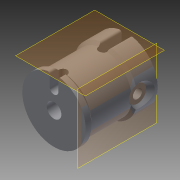
# Autodesk Inventor part: PULLEY
Saved by Autodesk Inventor 2013 (Build 170138000, 138)
## iProperties
Created: 2013-12-16
Part Number: PULLEY
Material: Generic
Document SubType Name: Modeling
Designer: employee
Density: 1 g/cm^3
Author: employee
Autodesk Inventor part; units mm, degrees
ref_plane "XY Plane" through (0, 0, 0) normal (0, 0, 1) x (1, 0, 0)
sketch "Sketch1" plane through (0, 0, 0) normal (0, 0, 1) x (1, 0, 0)
  circle A0 centre (0, 0) radius 10
  dimension "d0" = 20
  constraints: 1 centre point, 1 coincident
  measures "d0" diameter of A0
extrude "Extrusion1" add sketch "Sketch1" along normal blind 25
sketch "Sketch2" plane through (0, 0, 0) normal (0, 0, -1) x (-1, 0, 0)
  circle A0 centre (0, 0) radius 10 projected
  circle A1 centre (0, 0) radius 11
  dimension "d4" = 1
  constraints: 1 centre point, 1 coincident
  measures "d4" radial gap between concentric circles of A1 A0
extrude "Extrusion2" add sketch "Sketch2" against normal blind 8
sketch "Sketch3" plane through (0, 0, 25) normal (0, 0, 1) x (1, 0, 0)
  circle A0 centre (0, 0) radius 10 projected
  circle A1 centre (0, 0) radius 11
  dimension "d7" = 1
  constraints: 1 centre point, 1 coincident
  measures "d7" radial gap between concentric circles of A1 A0
extrude "Extrusion3" add sketch "Sketch3" against normal blind 3
chamfer "Chamfer1" distance 1 angle 45 1 edges at (-11, 0, 22)
sketch "Sketch4" plane through (0, 0, 0) normal (1, 0, 0) x (0, 1, 0)
  line L0 (-11, 0) -> (-11, 8) projected
  line L1 (-11, 8) -> (-10, 8) projected
  line L2 (-10, 8) -> (-10, 22) projected
  line L3 (-10, 22) -> (-11, 23) projected
  line L4 (-11, 23) -> (-11, 25) projected
  line L5 (-11, 25) -> (11, 25) projected
  line L6 (11, 25) -> (11, 23) projected
  line L7 (11, 23) -> (10, 22) projected
  line L8 (10, 22) -> (10, 8) projected
  line L9 (10, 8) -> (11, 8) projected
  line L10 (11, 8) -> (11, 0) projected
  line L11 (11, 0) -> (-11, 0) projected
  circle A0 centre (0, 5.5) radius 1.6
  point P0 (0, 0)
  point P1 (0, 0)
  dimension "d14" = 3.2
  dimension "d17" = 2.5
  constraints: 1 centre point, 1 midpoint, 1 vertical alignment
  measures "d14" diameter of A0
  measures "d17" distance from line of L9 A0.centre
extrude "Extrusion4" cut sketch "Sketch4" along normal through all both and the other way through all contours A0
sketch "Sketch5" plane through (0, 0, 0) normal (0, 0, -1) x (-1, 0, 0)
  circle A0 centre (0, 0) radius 11 projected
  circle A1 centre (0, 0) radius 2.55
  circle A2 centre (0, 6.25) radius 1.5
  dimension "d20" = 5.1
  dimension "d22" = 6.25
  dimension "d23" = 3
  constraints: 2 centre point, 1 coincident, 1 vertical alignment
  measures "d20" diameter of A1
  measures "d22" distance of A2.centre A0.centre
  measures "d23" diameter of A2
extrude "Extrusion5" cut sketch "Sketch5" against normal through all contours A1 | A2
ref_plane "Work Plane1" through (0, 11, 25) normal (0, 1, 0) x (-1, 0, 0)
sketch "Sketch6" plane through (0, 11, 25) normal (0, 1, 0) x (-1, 0, 0)
  line L0 (-1.5, 0) -> (1.5, 0) projected
  line L1 (1.5, -25) -> (-1.5, -25) projected
  line L2 (11, -17) -> (-11, -17) projected
  line L3 (-10, -3) -> (10, -3) projected
  circle A0 centre (0, -17) radius 1.5
  circle A1 centre (0, -3) radius 1.5
  point P0 (0, -25)
  dimension "d26" = 3
  constraints: 2 centre point, 2 midpoint, 1 equal radius
  measures "d26" diameter of A0
extrude "Extrusion6" cut sketch "Sketch6" against normal up to surface round surface about axis through (0, 6.25, 0) along (0, 0, 1) radius 1.5 far side no
sketch "Sketch7" plane through (0, 0, 0) normal (0, 0, -1) x (-1, 0, 0)
  circle A0 centre (0, 6.25) radius 1.5 projected
  circle A1 centre (0, 0) radius 11 projected
  line L0 (-1.5, 6.25) -> (-1.5, 10.8972)
  line L1 (1.5, 6.25) -> (1.5, 10.8972)
  constraints: 4 end point, 4 point on circle, 2 tangent, 1 parallel, 1 vertical
extrude "Extrusion7" cut sketch "Sketch7" against normal up to next contours A0 L0 A1 L1 picked at (0.8444, 9.8461)
sketch "Sketch8" plane through (0, 0, 25) normal (0, 0, 1) x (1, 0, 0)
  circle A0 centre (0, 0) radius 11 projected
  circle A1 centre (0, 6.25) radius 1.5 projected
  line L0 (-1.5, 6.25) -> (-1.5, 10.8972)
  line L1 (1.5, 6.25) -> (1.5, 10.8972)
  constraints: 4 end point, 4 point on circle, 2 tangent, 1 parallel, 1 vertical
extrude "Extrusion8" cut sketch "Sketch8" against normal up to next contours L1 A1 L0 A0 picked at (0.8444, 9.8461)
chamfer "Chamfer2" distance 1 angle 45 1 edges at (0, -11, 8)
sketch "Sketch9" plane through (0, 0, 0) normal (0, 0, -1) x (-1, 0, 0)
  circle A0 centre (0, 0) radius 2.55 projected
  line L0 (-7.55, -2.8) -> (-3.55, -2.8)
  line L1 (-3.55, -2.8) -> (-3.55, 2.8)
  line L2 (-3.55, 2.8) -> (-7.55, 2.8)
  line L3 (-7.55, 2.8) -> (-7.55, -2.8)
  line L4 (3.55, -2.8) -> (7.55, -2.8)
  line L5 (7.55, -2.8) -> (7.55, 2.8)
  line L6 (7.55, 2.8) -> (3.55, 2.8)
  line L7 (3.55, 2.8) -> (3.55, -2.8)
  line L8 (-2.55, 0) -> (-3.55, 0)
  line L9 (3.55, 0) -> (2.55, 0)
  dimension "d38" = 4
  dimension "d40" = 5.6
  dimension "d41" = 1
  constraints: 20 end point, 8 equal length, 3 horizontal alignment, 2 horizontal, 2 midpoint, 2 perpendicular, 2 point on circle
  measures "d38" distance of L1.end L2.end
  measures "d40" distance of L0.end L1.end
  measures "d41" distance of L8.start L8.end
extrude "Extrusion9" cut sketch "Sketch9" against normal blind 5.5 contours L3 L2 L1 L0 | L7 L6 L5 L4
sketch "Sketch10" plane through (3.55, -2.8, 0) normal (1, 0, 0) x (0, 0, -1)
  arc A0 (-5.5, 1.2) -> (-5.5, 4.4) centre (-5.5, 2.8) ccw projected
  line L0 (0, 5.6) -> (-5.5, 5.6) projected
  line L1 (-8.7332, 2.8) -> (-7.1166, 5.6)
  line L2 (-7.1166, 5.6) -> (-3.8834, 5.6)
  line L3 (-3.8834, 5.6) -> (-2.2668, 2.8)
  line L4 (-2.2668, 2.8) -> (-3.8834, 0)
  line L5 (-3.8834, 0) -> (-7.1166, 0)
  line L6 (-7.1166, 0) -> (-8.7332, 2.8)
  point P0 (0, 2.8)
  constraints: 12 end point, 1 coincident, 1 collinear, 1 midpoint, 13 other
extrude "Extrusion10" cut sketch "Sketch10" along normal up to surface (4 mm away)
pattern_circular "Circular Pattern1" count 2 over 360 about axis through (0, 0, 0) along (0, 0, 1) of "Extrusion10"
fillet "Fillet1" radius 0.75 4 edges at (1.5, 10.8972, 3.5) (-1.5, 10.8972, 3.5) (-1.5, 10.8972, 23.9999) (1.5, 10.8972, 23.9999)
ref_plane "Work Plane2" through (9.5, 0, 0) normal (1, 0, 0) x (0, 1, 0)
sketch "Sketch15" plane through (9.5, 0, 0) normal (1, 0, 0) x (0, 1, 0)
  line L0 (-3.1225, 8) -> (-3.1225, 22) projected
  line L1 (-5.5453, 23) -> (-5.5453, 25) projected
  line L2 (-5.5453, 25) -> (5.5453, 25) projected
  line L3 (5.5453, 25) -> (5.5453, 23) projected
  line L4 (3.1225, 22) -> (3.1225, 8) projected
  line L5 (5.5453, 7) -> (5.5453, 0) projected
  line L6 (5.5453, 0) -> (-5.5453, 0) projected
  line L7 (-5.5453, 0) -> (-5.5453, 7) projected
  circle A0 centre (0, 5.5) radius 1.6 projected
  circle A1 centre (0, 5.5) radius 3
  point P0 (0, 0)
  dimension "d64" = 6
  constraints: 1 centre point, 1 coincident, 4 other
  measures "d64" diameter of A1
extrude "Extrusion15" cut sketch "Sketch15" along normal blind 25.4 draft 45 contours A0 | A1
pattern_circular "Circular Pattern3" count 2 over 360 about axis through (0, 0, 0) along (0, 0, 1) of "Extrusion15"
fillet "Fillet3" radius 1 8 edges at (7.55, 0, 0) (5.55, 2.8, 0) (3.55, 0, 0) (5.55, -2.8, 0) (-3.55, 0, 0) (-7.55, 0, 0) (-5.55, 2.8, 0) (-5.55, -2.8, 0)
sketch "Sketch11" plane through (0, 0, 0) normal (0, 0, -1) x (-1, 0, 0)
  arc A0 (-2.4146, 10.7317) -> (2.4146, 10.7317) centre (0, 0) ccw projected
  line L0 (7.55, 2.8) -> (7.55, -2.8) projected
  line L1 (-9.5, 5.5453) -> (-9.5, -5.5453)
  line L2 (9.5, -5.5453) -> (9.5, 5.5453)
  dimension "d50" = 9.5
  constraints: 4 end point, 4 point on circle, 3 parallel
  measures "d50" distance from line of L2 A0.centre
sketch "Sketch14" plane through (-9.5, -5.5453, 0) normal (-1, 0, 0) x (0, 0, 1)
  line L0 (0, 11.0905) -> (7, 11.0905) projected
  line L1 (0, 0) -> (0, 11.0905) projected
  line L2 (7, 0) -> (0, 0) projected
  point P0 (0, 5.5453)
  constraints: 1 vertical alignment, 2 other
body "Solid1"
